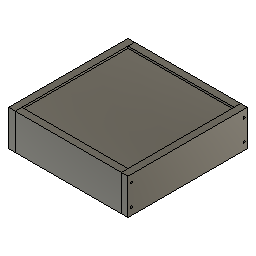
frame_16x16 (Autodesk Fusion 360 design; units mm, degrees)
Autodesk Fusion 360 part; units mm, degrees
note: some values were not read from the file. Set by a fixed rule: which sketch regions a step uses.
(part 1 of 4)
sketch "Sketch1" plane through (0, 0, 0) normal (0, 0, 1) x (1, 0, 0) in component "LED_Pannel"
  line L0 (0, 0) -> (160, 0)
  line L1 (160, 0) -> (160, 160)
  line L2 (160, 160) -> (0, 160)
  line L3 (0, 160) -> (0, 0)
  dimension "d1" = 160
  dimension "d2" = 160
  constraint horizontal L0
  constraint vertical L1
  constraint horizontal L2
  constraint vertical L3
  constraint coincident L0.start L3.end
  measures "d1" distance of L0.start L0.end
  measures "d2" distance of L0.start L2.end
extrude "Extrude1" add sketch "Sketch1" along normal blind 0.2 makes body 1 in component "LED_Pannel"
sketch "Sketch2" plane through (0, 0, 0.2) normal (0, 0, 1) x (-1, 0, 0) in component "LED_Pannel"
  line L0 (0, -160) -> (0, 0)
  line L1 (0, 0) -> (-160, 0)
  line L2 (-160, 0) -> (-160, -160)
  line L3 (-160, -160) -> (0, -160)
  line L4 (-2.5, -2.5) -> (-7.5, -2.5)
  line L5 (-7.5, -2.5) -> (-7.5, -7.5)
  line L6 (-7.5, -7.5) -> (-2.5, -7.5)
  line L7 (-2.5, -7.5) -> (-2.5, -2.5)
  line L8 (-12.5, -7.5) -> (-12.5, -2.5)
  line L9 (-17.5, -7.5) -> (-12.5, -7.5)
  line L10 (-17.5, -2.5) -> (-17.5, -7.5)
  line L11 (-12.5, -2.5) -> (-17.5, -2.5)
  line L12 (-22.5, -7.5) -> (-22.5, -2.5)
  line L13 (-27.5, -7.5) -> (-22.5, -7.5)
  line L14 (-27.5, -2.5) -> (-27.5, -7.5)
  line L15 (-22.5, -2.5) -> (-27.5, -2.5)
  line L16 (-32.5, -7.5) -> (-32.5, -2.5)
  line L17 (-37.5, -7.5) -> (-32.5, -7.5)
  line L18 (-37.5, -2.5) -> (-37.5, -7.5)
  line L19 (-32.5, -2.5) -> (-37.5, -2.5)
  line L20 (-42.5, -7.5) -> (-42.5, -2.5)
  line L21 (-47.5, -7.5) -> (-42.5, -7.5)
  line L22 (-47.5, -2.5) -> (-47.5, -7.5)
  line L23 (-42.5, -2.5) -> (-47.5, -2.5)
  line L24 (-52.5, -7.5) -> (-52.5, -2.5)
  line L25 (-57.5, -7.5) -> (-52.5, -7.5)
  line L26 (-57.5, -2.5) -> (-57.5, -7.5)
  line L27 (-52.5, -2.5) -> (-57.5, -2.5)
  line L28 (-62.5, -7.5) -> (-62.5, -2.5)
  line L29 (-67.5, -7.5) -> (-62.5, -7.5)
  line L30 (-67.5, -2.5) -> (-67.5, -7.5)
  line L31 (-62.5, -2.5) -> (-67.5, -2.5)
  line L32 (-72.5, -7.5) -> (-72.5, -2.5)
  line L33 (-77.5, -7.5) -> (-72.5, -7.5)
  line L34 (-77.5, -2.5) -> (-77.5, -7.5)
  line L35 (-72.5, -2.5) -> (-77.5, -2.5)
  line L36 (-82.5, -7.5) -> (-82.5, -2.5)
  line L37 (-87.5, -7.5) -> (-82.5, -7.5)
  line L38 (-87.5, -2.5) -> (-87.5, -7.5)
  line L39 (-82.5, -2.5) -> (-87.5, -2.5)
  line L40 (-92.5, -7.5) -> (-92.5, -2.5)
  line L41 (-97.5, -7.5) -> (-92.5, -7.5)
  line L42 (-97.5, -2.5) -> (-97.5, -7.5)
  line L43 (-92.5, -2.5) -> (-97.5, -2.5)
  line L44 (-102.5, -7.5) -> (-102.5, -2.5)
  line L45 (-107.5, -7.5) -> (-102.5, -7.5)
  line L46 (-107.5, -2.5) -> (-107.5, -7.5)
  line L47 (-102.5, -2.5) -> (-107.5, -2.5)
  line L48 (-112.5, -7.5) -> (-112.5, -2.5)
  line L49 (-117.5, -7.5) -> (-112.5, -7.5)
  line L50 (-117.5, -2.5) -> (-117.5, -7.5)
  line L51 (-112.5, -2.5) -> (-117.5, -2.5)
  line L52 (-122.5, -7.5) -> (-122.5, -2.5)
  line L53 (-127.5, -7.5) -> (-122.5, -7.5)
  line L54 (-127.5, -2.5) -> (-127.5, -7.5)
  line L55 (-122.5, -2.5) -> (-127.5, -2.5)
  line L56 (-132.5, -7.5) -> (-132.5, -2.5)
  line L57 (-137.5, -7.5) -> (-132.5, -7.5)
  line L58 (-137.5, -2.5) -> (-137.5, -7.5)
  line L59 (-132.5, -2.5) -> (-137.5, -2.5)
  line L60 (-142.5, -7.5) -> (-142.5, -2.5)
  line L61 (-147.5, -7.5) -> (-142.5, -7.5)
  line L62 (-147.5, -2.5) -> (-147.5, -7.5)
  line L63 (-142.5, -2.5) -> (-147.5, -2.5)
  line L64 (-152.5, -7.5) -> (-152.5, -2.5)
  line L65 (-157.5, -7.5) -> (-152.5, -7.5)
  line L66 (-157.5, -2.5) -> (-157.5, -7.5)
  line L67 (-152.5, -2.5) -> (-157.5, -2.5)
  line L68 (-2.5, -17.5) -> (-2.5, -12.5)
  line L69 (-7.5, -17.5) -> (-2.5, -17.5)
  line L70 (-7.5, -12.5) -> (-7.5, -17.5)
  line L71 (-2.5, -12.5) -> (-7.5, -12.5)
  line L72 (-12.5, -17.5) -> (-12.5, -12.5)
  line L73 (-17.5, -17.5) -> (-12.5, -17.5)
  line L74 (-17.5, -12.5) -> (-17.5, -17.5)
  line L75 (-12.5, -12.5) -> (-17.5, -12.5)
  line L76 (-22.5, -17.5) -> (-22.5, -12.5)
  line L77 (-27.5, -17.5) -> (-22.5, -17.5)
  line L78 (-27.5, -12.5) -> (-27.5, -17.5)
  line L79 (-22.5, -12.5) -> (-27.5, -12.5)
  line L80 (-32.5, -17.5) -> (-32.5, -12.5)
  line L81 (-37.5, -17.5) -> (-32.5, -17.5)
  line L82 (-37.5, -12.5) -> (-37.5, -17.5)
  line L83 (-32.5, -12.5) -> (-37.5, -12.5)
  line L84 (-42.5, -17.5) -> (-42.5, -12.5)
  line L85 (-47.5, -17.5) -> (-42.5, -17.5)
  line L86 (-47.5, -12.5) -> (-47.5, -17.5)
  line L87 (-42.5, -12.5) -> (-47.5, -12.5)
  line L88 (-52.5, -17.5) -> (-52.5, -12.5)
  line L89 (-57.5, -17.5) -> (-52.5, -17.5)
  line L90 (-57.5, -12.5) -> (-57.5, -17.5)
  line L91 (-52.5, -12.5) -> (-57.5, -12.5)
  line L92 (-62.5, -17.5) -> (-62.5, -12.5)
  line L93 (-67.5, -17.5) -> (-62.5, -17.5)
  line L94 (-67.5, -12.5) -> (-67.5, -17.5)
  line L95 (-62.5, -12.5) -> (-67.5, -12.5)
  line L96 (-72.5, -17.5) -> (-72.5, -12.5)
  line L97 (-77.5, -17.5) -> (-72.5, -17.5)
  line L98 (-77.5, -12.5) -> (-77.5, -17.5)
  line L99 (-72.5, -12.5) -> (-77.5, -12.5)
  line L100 (-82.5, -17.5) -> (-82.5, -12.5)
  line L101 (-87.5, -17.5) -> (-82.5, -17.5)
  line L102 (-87.5, -12.5) -> (-87.5, -17.5)
  line L103 (-82.5, -12.5) -> (-87.5, -12.5)
  line L104 (-92.5, -17.5) -> (-92.5, -12.5)
  line L105 (-97.5, -17.5) -> (-92.5, -17.5)
  line L106 (-97.5, -12.5) -> (-97.5, -17.5)
  line L107 (-92.5, -12.5) -> (-97.5, -12.5)
  line L108 (-102.5, -17.5) -> (-102.5, -12.5)
  line L109 (-107.5, -17.5) -> (-102.5, -17.5)
  line L110 (-107.5, -12.5) -> (-107.5, -17.5)
  line L111 (-102.5, -12.5) -> (-107.5, -12.5)
  line L112 (-112.5, -17.5) -> (-112.5, -12.5)
  line L113 (-117.5, -17.5) -> (-112.5, -17.5)
  line L114 (-117.5, -12.5) -> (-117.5, -17.5)
  line L115 (-112.5, -12.5) -> (-117.5, -12.5)
  line L116 (-122.5, -17.5) -> (-122.5, -12.5)
  line L117 (-127.5, -17.5) -> (-122.5, -17.5)
  line L118 (-127.5, -12.5) -> (-127.5, -17.5)
  line L119 (-122.5, -12.5) -> (-127.5, -12.5)
  line L120 (-132.5, -17.5) -> (-132.5, -12.5)
  line L121 (-137.5, -17.5) -> (-132.5, -17.5)
  line L122 (-137.5, -12.5) -> (-137.5, -17.5)
  line L123 (-132.5, -12.5) -> (-137.5, -12.5)
  line L124 (-142.5, -17.5) -> (-142.5, -12.5)
  line L125 (-147.5, -17.5) -> (-142.5, -17.5)
  line L126 (-147.5, -12.5) -> (-147.5, -17.5)
  line L127 (-142.5, -12.5) -> (-147.5, -12.5)
  line L128 (-152.5, -17.5) -> (-152.5, -12.5)
  line L129 (-157.5, -17.5) -> (-152.5, -17.5)
  line L130 (-157.5, -12.5) -> (-157.5, -17.5)
  line L131 (-152.5, -12.5) -> (-157.5, -12.5)
  line L132 (-2.5, -27.5) -> (-2.5, -22.5)
  line L133 (-7.5, -27.5) -> (-2.5, -27.5)
  line L134 (-7.5, -22.5) -> (-7.5, -27.5)
  line L135 (-2.5, -22.5) -> (-7.5, -22.5)
  line L136 (-12.5, -27.5) -> (-12.5, -22.5)
  line L137 (-17.5, -27.5) -> (-12.5, -27.5)
  line L138 (-17.5, -22.5) -> (-17.5, -27.5)
  line L139 (-12.5, -22.5) -> (-17.5, -22.5)
  line L140 (-22.5, -27.5) -> (-22.5, -22.5)
  line L141 (-27.5, -27.5) -> (-22.5, -27.5)
  line L142 (-27.5, -22.5) -> (-27.5, -27.5)
  line L143 (-22.5, -22.5) -> (-27.5, -22.5)
  line L144 (-32.5, -27.5) -> (-32.5, -22.5)
  line L145 (-37.5, -27.5) -> (-32.5, -27.5)
  line L146 (-37.5, -22.5) -> (-37.5, -27.5)
  line L147 (-32.5, -22.5) -> (-37.5, -22.5)
  line L148 (-42.5, -27.5) -> (-42.5, -22.5)
  line L149 (-47.5, -27.5) -> (-42.5, -27.5)
  line L150 (-47.5, -22.5) -> (-47.5, -27.5)
  line L151 (-42.5, -22.5) -> (-47.5, -22.5)
  line L152 (-52.5, -27.5) -> (-52.5, -22.5)
  line L153 (-57.5, -27.5) -> (-52.5, -27.5)
  line L154 (-57.5, -22.5) -> (-57.5, -27.5)
  line L155 (-52.5, -22.5) -> (-57.5, -22.5)
  line L156 (-62.5, -27.5) -> (-62.5, -22.5)
  line L157 (-67.5, -27.5) -> (-62.5, -27.5)
  line L158 (-67.5, -22.5) -> (-67.5, -27.5)
  line L159 (-62.5, -22.5) -> (-67.5, -22.5)
  line L160 (-72.5, -27.5) -> (-72.5, -22.5)
  line L161 (-77.5, -27.5) -> (-72.5, -27.5)
  line L162 (-77.5, -22.5) -> (-77.5, -27.5)
  line L163 (-72.5, -22.5) -> (-77.5, -22.5)
  line L164 (-82.5, -27.5) -> (-82.5, -22.5)
  line L165 (-87.5, -27.5) -> (-82.5, -27.5)
  line L166 (-87.5, -22.5) -> (-87.5, -27.5)
  line L167 (-82.5, -22.5) -> (-87.5, -22.5)
  line L168 (-92.5, -27.5) -> (-92.5, -22.5)
  line L169 (-97.5, -27.5) -> (-92.5, -27.5)
  line L170 (-97.5, -22.5) -> (-97.5, -27.5)
  line L171 (-92.5, -22.5) -> (-97.5, -22.5)
  line L172 (-102.5, -27.5) -> (-102.5, -22.5)
  line L173 (-107.5, -27.5) -> (-102.5, -27.5)
  line L174 (-107.5, -22.5) -> (-107.5, -27.5)
  line L175 (-102.5, -22.5) -> (-107.5, -22.5)
  line L176 (-112.5, -27.5) -> (-112.5, -22.5)
  line L177 (-117.5, -27.5) -> (-112.5, -27.5)
  line L178 (-117.5, -22.5) -> (-117.5, -27.5)
  line L179 (-112.5, -22.5) -> (-117.5, -22.5)
  line L180 (-122.5, -27.5) -> (-122.5, -22.5)
  line L181 (-127.5, -27.5) -> (-122.5, -27.5)
  line L182 (-127.5, -22.5) -> (-127.5, -27.5)
  line L183 (-122.5, -22.5) -> (-127.5, -22.5)
  line L184 (-132.5, -27.5) -> (-132.5, -22.5)
  line L185 (-137.5, -27.5) -> (-132.5, -27.5)
  line L186 (-137.5, -22.5) -> (-137.5, -27.5)
  line L187 (-132.5, -22.5) -> (-137.5, -22.5)
  line L188 (-142.5, -27.5) -> (-142.5, -22.5)
  line L189 (-147.5, -27.5) -> (-142.5, -27.5)
  line L190 (-147.5, -22.5) -> (-147.5, -27.5)
  line L191 (-142.5, -22.5) -> (-147.5, -22.5)
  line L192 (-152.5, -27.5) -> (-152.5, -22.5)
  line L193 (-157.5, -27.5) -> (-152.5, -27.5)
  line L194 (-157.5, -22.5) -> (-157.5, -27.5)
  line L195 (-152.5, -22.5) -> (-157.5, -22.5)
  line L196 (-2.5, -37.5) -> (-2.5, -32.5)
  line L197 (-7.5, -37.5) -> (-2.5, -37.5)
  line L198 (-7.5, -32.5) -> (-7.5, -37.5)
  line L199 (-2.5, -32.5) -> (-7.5, -32.5)
  line L200 (-12.5, -37.5) -> (-12.5, -32.5)
  line L201 (-17.5, -37.5) -> (-12.5, -37.5)
  line L202 (-17.5, -32.5) -> (-17.5, -37.5)
  line L203 (-12.5, -32.5) -> (-17.5, -32.5)
  line L204 (-22.5, -37.5) -> (-22.5, -32.5)
  line L205 (-27.5, -37.5) -> (-22.5, -37.5)
  line L206 (-27.5, -32.5) -> (-27.5, -37.5)
  line L207 (-22.5, -32.5) -> (-27.5, -32.5)
  line L208 (-32.5, -37.5) -> (-32.5, -32.5)
  line L209 (-37.5, -37.5) -> (-32.5, -37.5)
  line L210 (-37.5, -32.5) -> (-37.5, -37.5)
  line L211 (-32.5, -32.5) -> (-37.5, -32.5)
  line L212 (-42.5, -37.5) -> (-42.5, -32.5)
  line L213 (-47.5, -37.5) -> (-42.5, -37.5)
  line L214 (-47.5, -32.5) -> (-47.5, -37.5)
  line L215 (-42.5, -32.5) -> (-47.5, -32.5)
  line L216 (-52.5, -37.5) -> (-52.5, -32.5)
  line L217 (-57.5, -37.5) -> (-52.5, -37.5)
  line L218 (-57.5, -32.5) -> (-57.5, -37.5)
  line L219 (-52.5, -32.5) -> (-57.5, -32.5)
  line L220 (-62.5, -37.5) -> (-62.5, -32.5)
  line L221 (-67.5, -37.5) -> (-62.5, -37.5)
  line L222 (-67.5, -32.5) -> (-67.5, -37.5)
  line L223 (-62.5, -32.5) -> (-67.5, -32.5)
  line L224 (-72.5, -37.5) -> (-72.5, -32.5)
  line L225 (-77.5, -37.5) -> (-72.5, -37.5)
  line L226 (-77.5, -32.5) -> (-77.5, -37.5)
  line L227 (-72.5, -32.5) -> (-77.5, -32.5)
  line L228 (-82.5, -37.5) -> (-82.5, -32.5)
  line L229 (-87.5, -37.5) -> (-82.5, -37.5)
  line L230 (-87.5, -32.5) -> (-87.5, -37.5)
  line L231 (-82.5, -32.5) -> (-87.5, -32.5)
  line L232 (-92.5, -37.5) -> (-92.5, -32.5)
  line L233 (-97.5, -37.5) -> (-92.5, -37.5)
  line L234 (-97.5, -32.5) -> (-97.5, -37.5)
  line L235 (-92.5, -32.5) -> (-97.5, -32.5)
  line L236 (-102.5, -37.5) -> (-102.5, -32.5)
  line L237 (-107.5, -37.5) -> (-102.5, -37.5)
  line L238 (-107.5, -32.5) -> (-107.5, -37.5)
  line L239 (-102.5, -32.5) -> (-107.5, -32.5)
  line L240 (-112.5, -37.5) -> (-112.5, -32.5)
  line L241 (-117.5, -37.5) -> (-112.5, -37.5)
  line L242 (-117.5, -32.5) -> (-117.5, -37.5)
  line L243 (-112.5, -32.5) -> (-117.5, -32.5)
  line L244 (-122.5, -37.5) -> (-122.5, -32.5)
  line L245 (-127.5, -37.5) -> (-122.5, -37.5)
  line L246 (-127.5, -32.5) -> (-127.5, -37.5)
  line L247 (-122.5, -32.5) -> (-127.5, -32.5)
  line L248 (-132.5, -37.5) -> (-132.5, -32.5)
  line L249 (-137.5, -37.5) -> (-132.5, -37.5)
  line L250 (-137.5, -32.5) -> (-137.5, -37.5)
  line L251 (-132.5, -32.5) -> (-137.5, -32.5)
  line L252 (-142.5, -37.5) -> (-142.5, -32.5)
  line L253 (-147.5, -37.5) -> (-142.5, -37.5)
  line L254 (-147.5, -32.5) -> (-147.5, -37.5)
  line L255 (-142.5, -32.5) -> (-147.5, -32.5)
  line L256 (-152.5, -37.5) -> (-152.5, -32.5)
  line L257 (-157.5, -37.5) -> (-152.5, -37.5)
  line L258 (-157.5, -32.5) -> (-157.5, -37.5)
  line L259 (-152.5, -32.5) -> (-157.5, -32.5)
  line L260 (-2.5, -47.5) -> (-2.5, -42.5)
  line L261 (-7.5, -47.5) -> (-2.5, -47.5)
  line L262 (-7.5, -42.5) -> (-7.5, -47.5)
  line L263 (-2.5, -42.5) -> (-7.5, -42.5)
  line L264 (-12.5, -47.5) -> (-12.5, -42.5)
  line L265 (-17.5, -47.5) -> (-12.5, -47.5)
  line L266 (-17.5, -42.5) -> (-17.5, -47.5)
  line L267 (-12.5, -42.5) -> (-17.5, -42.5)
  line L268 (-22.5, -47.5) -> (-22.5, -42.5)
  line L269 (-27.5, -47.5) -> (-22.5, -47.5)
  line L270 (-27.5, -42.5) -> (-27.5, -47.5)
  line L271 (-22.5, -42.5) -> (-27.5, -42.5)
  line L272 (-32.5, -47.5) -> (-32.5, -42.5)
  line L273 (-37.5, -47.5) -> (-32.5, -47.5)
  line L274 (-37.5, -42.5) -> (-37.5, -47.5)
  line L275 (-32.5, -42.5) -> (-37.5, -42.5)
  line L276 (-42.5, -47.5) -> (-42.5, -42.5)
  line L277 (-47.5, -47.5) -> (-42.5, -47.5)
  line L278 (-47.5, -42.5) -> (-47.5, -47.5)
  line L279 (-42.5, -42.5) -> (-47.5, -42.5)
  line L280 (-52.5, -47.5) -> (-52.5, -42.5)
  line L281 (-57.5, -47.5) -> (-52.5, -47.5)
  line L282 (-57.5, -42.5) -> (-57.5, -47.5)
  line L283 (-52.5, -42.5) -> (-57.5, -42.5)
  line L284 (-62.5, -47.5) -> (-62.5, -42.5)
  line L285 (-67.5, -47.5) -> (-62.5, -47.5)
  line L286 (-67.5, -42.5) -> (-67.5, -47.5)
  line L287 (-62.5, -42.5) -> (-67.5, -42.5)
  line L288 (-72.5, -47.5) -> (-72.5, -42.5)
  line L289 (-77.5, -47.5) -> (-72.5, -47.5)
  line L290 (-77.5, -42.5) -> (-77.5, -47.5)
  line L291 (-72.5, -42.5) -> (-77.5, -42.5)
  line L292 (-82.5, -47.5) -> (-82.5, -42.5)
  line L293 (-87.5, -47.5) -> (-82.5, -47.5)
  line L294 (-87.5, -42.5) -> (-87.5, -47.5)
  line L295 (-82.5, -42.5) -> (-87.5, -42.5)
  line L296 (-92.5, -47.5) -> (-92.5, -42.5)
  line L297 (-97.5, -47.5) -> (-92.5, -47.5)
  line L298 (-97.5, -42.5) -> (-97.5, -47.5)
  line L299 (-92.5, -42.5) -> (-97.5, -42.5)
  line L300 (-102.5, -47.5) -> (-102.5, -42.5)
  line L301 (-107.5, -47.5) -> (-102.5, -47.5)
  line L302 (-107.5, -42.5) -> (-107.5, -47.5)
  line L303 (-102.5, -42.5) -> (-107.5, -42.5)
  line L304 (-112.5, -47.5) -> (-112.5, -42.5)
  line L305 (-117.5, -47.5) -> (-112.5, -47.5)
  line L306 (-117.5, -42.5) -> (-117.5, -47.5)
  line L307 (-112.5, -42.5) -> (-117.5, -42.5)
  line L308 (-122.5, -47.5) -> (-122.5, -42.5)
  line L309 (-127.5, -47.5) -> (-122.5, -47.5)
  line L310 (-127.5, -42.5) -> (-127.5, -47.5)
  line L311 (-122.5, -42.5) -> (-127.5, -42.5)
  line L312 (-132.5, -47.5) -> (-132.5, -42.5)
  line L313 (-137.5, -47.5) -> (-132.5, -47.5)
  line L314 (-137.5, -42.5) -> (-137.5, -47.5)
  line L315 (-132.5, -42.5) -> (-137.5, -42.5)
  line L316 (-142.5, -47.5) -> (-142.5, -42.5)
  line L317 (-147.5, -47.5) -> (-142.5, -47.5)
  line L318 (-147.5, -42.5) -> (-147.5, -47.5)
  line L319 (-142.5, -42.5) -> (-147.5, -42.5)
  line L320 (-152.5, -47.5) -> (-152.5, -42.5)
  line L321 (-157.5, -47.5) -> (-152.5, -47.5)
  line L322 (-157.5, -42.5) -> (-157.5, -47.5)
  line L323 (-152.5, -42.5) -> (-157.5, -42.5)
  line L324 (-2.5, -57.5) -> (-2.5, -52.5)
  line L325 (-7.5, -57.5) -> (-2.5, -57.5)
  line L326 (-7.5, -52.5) -> (-7.5, -57.5)
  line L327 (-2.5, -52.5) -> (-7.5, -52.5)
  line L328 (-12.5, -57.5) -> (-12.5, -52.5)
  line L329 (-17.5, -57.5) -> (-12.5, -57.5)
  line L330 (-17.5, -52.5) -> (-17.5, -57.5)
  line L331 (-12.5, -52.5) -> (-17.5, -52.5)
  line L332 (-22.5, -57.5) -> (-22.5, -52.5)
  line L333 (-27.5, -57.5) -> (-22.5, -57.5)
  line L334 (-27.5, -52.5) -> (-27.5, -57.5)
  line L335 (-22.5, -52.5) -> (-27.5, -52.5)
  line L336 (-32.5, -57.5) -> (-32.5, -52.5)
  line L337 (-37.5, -57.5) -> (-32.5, -57.5)
  line L338 (-37.5, -52.5) -> (-37.5, -57.5)
  line L339 (-32.5, -52.5) -> (-37.5, -52.5)
  line L340 (-42.5, -57.5) -> (-42.5, -52.5)
  line L341 (-47.5, -57.5) -> (-42.5, -57.5)
  line L342 (-47.5, -52.5) -> (-47.5, -57.5)
  line L343 (-42.5, -52.5) -> (-47.5, -52.5)
  line L344 (-52.5, -57.5) -> (-52.5, -52.5)
  line L345 (-57.5, -57.5) -> (-52.5, -57.5)
  line L346 (-57.5, -52.5) -> (-57.5, -57.5)
  line L347 (-52.5, -52.5) -> (-57.5, -52.5)
  line L348 (-62.5, -57.5) -> (-62.5, -52.5)
  line L349 (-67.5, -57.5) -> (-62.5, -57.5)
  line L350 (-67.5, -52.5) -> (-67.5, -57.5)
  line L351 (-62.5, -52.5) -> (-67.5, -52.5)
  line L352 (-72.5, -57.5) -> (-72.5, -52.5)
  line L353 (-77.5, -57.5) -> (-72.5, -57.5)
  line L354 (-77.5, -52.5) -> (-77.5, -57.5)
  line L355 (-72.5, -52.5) -> (-77.5, -52.5)
  line L356 (-82.5, -57.5) -> (-82.5, -52.5)
  line L357 (-87.5, -57.5) -> (-82.5, -57.5)
  line L358 (-87.5, -52.5) -> (-87.5, -57.5)
  line L359 (-82.5, -52.5) -> (-87.5, -52.5)
  line L360 (-92.5, -57.5) -> (-92.5, -52.5)
  line L361 (-97.5, -57.5) -> (-92.5, -57.5)
  line L362 (-97.5, -52.5) -> (-97.5, -57.5)
  line L363 (-92.5, -52.5) -> (-97.5, -52.5)
  line L364 (-102.5, -57.5) -> (-102.5, -52.5)
  line L365 (-107.5, -57.5) -> (-102.5, -57.5)
  line L366 (-107.5, -52.5) -> (-107.5, -57.5)
  line L367 (-102.5, -52.5) -> (-107.5, -52.5)
  line L368 (-112.5, -57.5) -> (-112.5, -52.5)
  line L369 (-117.5, -57.5) -> (-112.5, -57.5)
  line L370 (-117.5, -52.5) -> (-117.5, -57.5)
  line L371 (-112.5, -52.5) -> (-117.5, -52.5)
  line L372 (-122.5, -57.5) -> (-122.5, -52.5)
  line L373 (-127.5, -57.5) -> (-122.5, -57.5)
  line L374 (-127.5, -52.5) -> (-127.5, -57.5)
  line L375 (-122.5, -52.5) -> (-127.5, -52.5)
  line L376 (-132.5, -57.5) -> (-132.5, -52.5)
  line L377 (-137.5, -57.5) -> (-132.5, -57.5)
  line L378 (-137.5, -52.5) -> (-137.5, -57.5)
  line L379 (-132.5, -52.5) -> (-137.5, -52.5)
  line L380 (-142.5, -57.5) -> (-142.5, -52.5)
  line L381 (-147.5, -57.5) -> (-142.5, -57.5)
  line L382 (-147.5, -52.5) -> (-147.5, -57.5)
  line L383 (-142.5, -52.5) -> (-147.5, -52.5)
  line L384 (-152.5, -57.5) -> (-152.5, -52.5)
  line L385 (-157.5, -57.5) -> (-152.5, -57.5)
  line L386 (-157.5, -52.5) -> (-157.5, -57.5)
  line L387 (-152.5, -52.5) -> (-157.5, -52.5)
  line L388 (-2.5, -67.5) -> (-2.5, -62.5)
  line L389 (-7.5, -67.5) -> (-2.5, -67.5)
  line L390 (-7.5, -62.5) -> (-7.5, -67.5)
  line L391 (-2.5, -62.5) -> (-7.5, -62.5)
  line L392 (-12.5, -67.5) -> (-12.5, -62.5)
  line L393 (-17.5, -67.5) -> (-12.5, -67.5)
  line L394 (-17.5, -62.5) -> (-17.5, -67.5)
  line L395 (-12.5, -62.5) -> (-17.5, -62.5)
  line L396 (-22.5, -67.5) -> (-22.5, -62.5)
  line L397 (-27.5, -67.5) -> (-22.5, -67.5)
  line L398 (-27.5, -62.5) -> (-27.5, -67.5)
  line L399 (-22.5, -62.5) -> (-27.5, -62.5)
  line L400 (-32.5, -67.5) -> (-32.5, -62.5)
  line L401 (-37.5, -67.5) -> (-32.5, -67.5)
  line L402 (-37.5, -62.5) -> (-37.5, -67.5)
  line L403 (-32.5, -62.5) -> (-37.5, -62.5)
  line L404 (-42.5, -67.5) -> (-42.5, -62.5)
  line L405 (-47.5, -67.5) -> (-42.5, -67.5)
  line L406 (-47.5, -62.5) -> (-47.5, -67.5)
  line L407 (-42.5, -62.5) -> (-47.5, -62.5)
  line L408 (-52.5, -67.5) -> (-52.5, -62.5)
  line L409 (-57.5, -67.5) -> (-52.5, -67.5)
  line L410 (-57.5, -62.5) -> (-57.5, -67.5)
  line L411 (-52.5, -62.5) -> (-57.5, -62.5)
  line L412 (-62.5, -67.5) -> (-62.5, -62.5)
  line L413 (-67.5, -67.5) -> (-62.5, -67.5)
  line L414 (-67.5, -62.5) -> (-67.5, -67.5)
  line L415 (-62.5, -62.5) -> (-67.5, -62.5)
  line L416 (-72.5, -67.5) -> (-72.5, -62.5)
  line L417 (-77.5, -67.5) -> (-72.5, -67.5)
  line L418 (-77.5, -62.5) -> (-77.5, -67.5)
  line L419 (-72.5, -62.5) -> (-77.5, -62.5)
  line L420 (-82.5, -67.5) -> (-82.5, -62.5)
  line L421 (-87.5, -67.5) -> (-82.5, -67.5)
  line L422 (-87.5, -62.5) -> (-87.5, -67.5)
  line L423 (-82.5, -62.5) -> (-87.5, -62.5)
  line L424 (-92.5, -67.5) -> (-92.5, -62.5)
  line L425 (-97.5, -67.5) -> (-92.5, -67.5)
  line L426 (-97.5, -62.5) -> (-97.5, -67.5)
  line L427 (-92.5, -62.5) -> (-97.5, -62.5)
  line L428 (-102.5, -67.5) -> (-102.5, -62.5)
  line L429 (-107.5, -67.5) -> (-102.5, -67.5)
  line L430 (-107.5, -62.5) -> (-107.5, -67.5)
  line L431 (-102.5, -62.5) -> (-107.5, -62.5)
  line L432 (-112.5, -67.5) -> (-112.5, -62.5)
  line L433 (-117.5, -67.5) -> (-112.5, -67.5)
  line L434 (-117.5, -62.5) -> (-117.5, -67.5)
  line L435 (-112.5, -62.5) -> (-117.5, -62.5)
  line L436 (-122.5, -67.5) -> (-122.5, -62.5)
  line L437 (-127.5, -67.5) -> (-122.5, -67.5)
  line L438 (-127.5, -62.5) -> (-127.5, -67.5)
  line L439 (-122.5, -62.5) -> (-127.5, -62.5)
  line L440 (-132.5, -67.5) -> (-132.5, -62.5)
  line L441 (-137.5, -67.5) -> (-132.5, -67.5)
  line L442 (-137.5, -62.5) -> (-137.5, -67.5)
  line L443 (-132.5, -62.5) -> (-137.5, -62.5)
  line L444 (-142.5, -67.5) -> (-142.5, -62.5)
  line L445 (-147.5, -67.5) -> (-142.5, -67.5)
  line L446 (-147.5, -62.5) -> (-147.5, -67.5)
  line L447 (-142.5, -62.5) -> (-147.5, -62.5)
  line L448 (-152.5, -67.5) -> (-152.5, -62.5)
  line L449 (-157.5, -67.5) -> (-152.5, -67.5)
  line L450 (-157.5, -62.5) -> (-157.5, -67.5)
  line L451 (-152.5, -62.5) -> (-157.5, -62.5)
  line L452 (-2.5, -77.5) -> (-2.5, -72.5)
  line L453 (-7.5, -77.5) -> (-2.5, -77.5)
  line L454 (-7.5, -72.5) -> (-7.5, -77.5)
  line L455 (-2.5, -72.5) -> (-7.5, -72.5)
  line L456 (-12.5, -77.5) -> (-12.5, -72.5)
  line L457 (-17.5, -77.5) -> (-12.5, -77.5)
  line L458 (-17.5, -72.5) -> (-17.5, -77.5)
  line L459 (-12.5, -72.5) -> (-17.5, -72.5)
  line L460 (-22.5, -77.5) -> (-22.5, -72.5)
  line L461 (-27.5, -77.5) -> (-22.5, -77.5)
  line L462 (-27.5, -72.5) -> (-27.5, -77.5)
  line L463 (-22.5, -72.5) -> (-27.5, -72.5)
  line L464 (-32.5, -77.5) -> (-32.5, -72.5)
  line L465 (-37.5, -77.5) -> (-32.5, -77.5)
  line L466 (-37.5, -72.5) -> (-37.5, -77.5)
  line L467 (-32.5, -72.5) -> (-37.5, -72.5)
  line L468 (-42.5, -77.5) -> (-42.5, -72.5)
  line L469 (-47.5, -77.5) -> (-42.5, -77.5)
  line L470 (-47.5, -72.5) -> (-47.5, -77.5)
  line L471 (-42.5, -72.5) -> (-47.5, -72.5)
  line L472 (-52.5, -77.5) -> (-52.5, -72.5)
  line L473 (-57.5, -77.5) -> (-52.5, -77.5)
  line L474 (-57.5, -72.5) -> (-57.5, -77.5)
  line L475 (-52.5, -72.5) -> (-57.5, -72.5)
  line L476 (-62.5, -77.5) -> (-62.5, -72.5)
  line L477 (-67.5, -77.5) -> (-62.5, -77.5)
  line L478 (-67.5, -72.5) -> (-67.5, -77.5)
  line L479 (-62.5, -72.5) -> (-67.5, -72.5)
  line L480 (-72.5, -77.5) -> (-72.5, -72.5)
  line L481 (-77.5, -77.5) -> (-72.5, -77.5)
  line L482 (-77.5, -72.5) -> (-77.5, -77.5)
  line L483 (-72.5, -72.5) -> (-77.5, -72.5)
  line L484 (-82.5, -77.5) -> (-82.5, -72.5)
  line L485 (-87.5, -77.5) -> (-82.5, -77.5)
  line L486 (-87.5, -72.5) -> (-87.5, -77.5)
  line L487 (-82.5, -72.5) -> (-87.5, -72.5)
  line L488 (-92.5, -77.5) -> (-92.5, -72.5)
  line L489 (-97.5, -77.5) -> (-92.5, -77.5)
  line L490 (-97.5, -72.5) -> (-97.5, -77.5)
  line L491 (-92.5, -72.5) -> (-97.5, -72.5)
  line L492 (-102.5, -77.5) -> (-102.5, -72.5)
  line L493 (-107.5, -77.5) -> (-102.5, -77.5)
  line L494 (-107.5, -72.5) -> (-107.5, -77.5)
  line L495 (-102.5, -72.5) -> (-107.5, -72.5)
  line L496 (-112.5, -77.5) -> (-112.5, -72.5)
  line L497 (-117.5, -77.5) -> (-112.5, -77.5)
  line L498 (-117.5, -72.5) -> (-117.5, -77.5)
  line L499 (-112.5, -72.5) -> (-117.5, -72.5)
  line L500 (-122.5, -77.5) -> (-122.5, -72.5)
  line L501 (-127.5, -77.5) -> (-122.5, -77.5)
  line L502 (-127.5, -72.5) -> (-127.5, -77.5)
  line L503 (-122.5, -72.5) -> (-127.5, -72.5)
  line L504 (-132.5, -77.5) -> (-132.5, -72.5)
  line L505 (-137.5, -77.5) -> (-132.5, -77.5)
  line L506 (-137.5, -72.5) -> (-137.5, -77.5)
  line L507 (-132.5, -72.5) -> (-137.5, -72.5)
  line L508 (-142.5, -77.5) -> (-142.5, -72.5)
  line L509 (-147.5, -77.5) -> (-142.5, -77.5)
  line L510 (-147.5, -72.5) -> (-147.5, -77.5)
  line L511 (-142.5, -72.5) -> (-147.5, -72.5)
  line L512 (-152.5, -77.5) -> (-152.5, -72.5)
  line L513 (-157.5, -77.5) -> (-152.5, -77.5)
  line L514 (-157.5, -72.5) -> (-157.5, -77.5)
  line L515 (-152.5, -72.5) -> (-157.5, -72.5)
  line L516 (-2.5, -87.5) -> (-2.5, -82.5)
  line L517 (-7.5, -87.5) -> (-2.5, -87.5)
  line L518 (-7.5, -82.5) -> (-7.5, -87.5)
  line L519 (-2.5, -82.5) -> (-7.5, -82.5)
  line L520 (-12.5, -87.5) -> (-12.5, -82.5)
  line L521 (-17.5, -87.5) -> (-12.5, -87.5)
  line L522 (-17.5, -82.5) -> (-17.5, -87.5)
  line L523 (-12.5, -82.5) -> (-17.5, -82.5)
  line L524 (-22.5, -87.5) -> (-22.5, -82.5)
  line L525 (-27.5, -87.5) -> (-22.5, -87.5)
  line L526 (-27.5, -82.5) -> (-27.5, -87.5)
  line L527 (-22.5, -82.5) -> (-27.5, -82.5)
  line L528 (-32.5, -87.5) -> (-32.5, -82.5)
  line L529 (-37.5, -87.5) -> (-32.5, -87.5)
  line L530 (-37.5, -82.5) -> (-37.5, -87.5)
  line L531 (-32.5, -82.5) -> (-37.5, -82.5)
  line L532 (-42.5, -87.5) -> (-42.5, -82.5)
  line L533 (-47.5, -87.5) -> (-42.5, -87.5)
  line L534 (-47.5, -82.5) -> (-47.5, -87.5)
  line L535 (-42.5, -82.5) -> (-47.5, -82.5)
  line L536 (-52.5, -87.5) -> (-52.5, -82.5)
  line L537 (-57.5, -87.5) -> (-52.5, -87.5)
  line L538 (-57.5, -82.5) -> (-57.5, -87.5)
  line L539 (-52.5, -82.5) -> (-57.5, -82.5)
  line L540 (-62.5, -87.5) -> (-62.5, -82.5)
  line L541 (-67.5, -87.5) -> (-62.5, -87.5)
  line L542 (-67.5, -82.5) -> (-67.5, -87.5)
  line L543 (-62.5, -82.5) -> (-67.5, -82.5)
  line L544 (-72.5, -87.5) -> (-72.5, -82.5)
  line L545 (-77.5, -87.5) -> (-72.5, -87.5)
  line L546 (-77.5, -82.5) -> (-77.5, -87.5)
  line L547 (-72.5, -82.5) -> (-77.5, -82.5)
  line L548 (-82.5, -87.5) -> (-82.5, -82.5)
  line L549 (-87.5, -87.5) -> (-82.5, -87.5)
  line L550 (-87.5, -82.5) -> (-87.5, -87.5)
  line L551 (-82.5, -82.5) -> (-87.5, -82.5)
  line L552 (-92.5, -87.5) -> (-92.5, -82.5)
  line L553 (-97.5, -87.5) -> (-92.5, -87.5)
  line L554 (-97.5, -82.5) -> (-97.5, -87.5)
  line L555 (-92.5, -82.5) -> (-97.5, -82.5)
  line L556 (-102.5, -87.5) -> (-102.5, -82.5)
  line L557 (-107.5, -87.5) -> (-102.5, -87.5)
  line L558 (-107.5, -82.5) -> (-107.5, -87.5)
  line L559 (-102.5, -82.5) -> (-107.5, -82.5)
  line L560 (-112.5, -87.5) -> (-112.5, -82.5)
  line L561 (-117.5, -87.5) -> (-112.5, -87.5)
  line L562 (-117.5, -82.5) -> (-117.5, -87.5)
  line L563 (-112.5, -82.5) -> (-117.5, -82.5)
  line L564 (-122.5, -87.5) -> (-122.5, -82.5)
  line L565 (-127.5, -87.5) -> (-122.5, -87.5)
  line L566 (-127.5, -82.5) -> (-127.5, -87.5)
  line L567 (-122.5, -82.5) -> (-127.5, -82.5)
  line L568 (-132.5, -87.5) -> (-132.5, -82.5)
  line L569 (-137.5, -87.5) -> (-132.5, -87.5)
  line L570 (-137.5, -82.5) -> (-137.5, -87.5)
  line L571 (-132.5, -82.5) -> (-137.5, -82.5)
  line L572 (-142.5, -87.5) -> (-142.5, -82.5)
  line L573 (-147.5, -87.5) -> (-142.5, -87.5)
  line L574 (-147.5, -82.5) -> (-147.5, -87.5)
  line L575 (-142.5, -82.5) -> (-147.5, -82.5)
  line L576 (-152.5, -87.5) -> (-152.5, -82.5)
  line L577 (-157.5, -87.5) -> (-152.5, -87.5)
  line L578 (-157.5, -82.5) -> (-157.5, -87.5)
  line L579 (-152.5, -82.5) -> (-157.5, -82.5)
  line L580 (-2.5, -97.5) -> (-2.5, -92.5)
  line L581 (-7.5, -97.5) -> (-2.5, -97.5)
  line L582 (-7.5, -92.5) -> (-7.5, -97.5)
  line L583 (-2.5, -92.5) -> (-7.5, -92.5)
  line L584 (-12.5, -97.5) -> (-12.5, -92.5)
  line L585 (-17.5, -97.5) -> (-12.5, -97.5)
  line L586 (-17.5, -92.5) -> (-17.5, -97.5)
  line L587 (-12.5, -92.5) -> (-17.5, -92.5)
  line L588 (-22.5, -97.5) -> (-22.5, -92.5)
  line L589 (-27.5, -97.5) -> (-22.5, -97.5)
  line L590 (-27.5, -92.5) -> (-27.5, -97.5)
  line L591 (-22.5, -92.5) -> (-27.5, -92.5)
  line L592 (-32.5, -97.5) -> (-32.5, -92.5)
  line L593 (-37.5, -97.5) -> (-32.5, -97.5)
  line L594 (-37.5, -92.5) -> (-37.5, -97.5)
  line L595 (-32.5, -92.5) -> (-37.5, -92.5)
  line L596 (-42.5, -97.5) -> (-42.5, -92.5)
  line L597 (-47.5, -97.5) -> (-42.5, -97.5)
  line L598 (-47.5, -92.5) -> (-47.5, -97.5)
  line L599 (-42.5, -92.5) -> (-47.5, -92.5)
  line L600 (-52.5, -97.5) -> (-52.5, -92.5)
  line L601 (-57.5, -97.5) -> (-52.5, -97.5)
  line L602 (-57.5, -92.5) -> (-57.5, -97.5)
  line L603 (-52.5, -92.5) -> (-57.5, -92.5)
  line L604 (-62.5, -97.5) -> (-62.5, -92.5)
  line L605 (-67.5, -97.5) -> (-62.5, -97.5)
  line L606 (-67.5, -92.5) -> (-67.5, -97.5)
  line L607 (-62.5, -92.5) -> (-67.5, -92.5)
  line L608 (-72.5, -97.5) -> (-72.5, -92.5)
  line L609 (-77.5, -97.5) -> (-72.5, -97.5)
  line L610 (-77.5, -92.5) -> (-77.5, -97.5)
  line L611 (-72.5, -92.5) -> (-77.5, -92.5)
  line L612 (-82.5, -97.5) -> (-82.5, -92.5)
  line L613 (-87.5, -97.5) -> (-82.5, -97.5)
  line L614 (-87.5, -92.5) -> (-87.5, -97.5)
  line L615 (-82.5, -92.5) -> (-87.5, -92.5)
  line L616 (-92.5, -97.5) -> (-92.5, -92.5)
  line L617 (-97.5, -97.5) -> (-92.5, -97.5)
  line L618 (-97.5, -92.5) -> (-97.5, -97.5)
  line L619 (-92.5, -92.5) -> (-97.5, -92.5)
  line L620 (-102.5, -97.5) -> (-102.5, -92.5)
  line L621 (-107.5, -97.5) -> (-102.5, -97.5)
  line L622 (-107.5, -92.5) -> (-107.5, -97.5)
  line L623 (-102.5, -92.5) -> (-107.5, -92.5)
  line L624 (-112.5, -97.5) -> (-112.5, -92.5)
  line L625 (-117.5, -97.5) -> (-112.5, -97.5)
  line L626 (-117.5, -92.5) -> (-117.5, -97.5)
  line L627 (-112.5, -92.5) -> (-117.5, -92.5)
  line L628 (-122.5, -97.5) -> (-122.5, -92.5)
  line L629 (-127.5, -97.5) -> (-122.5, -97.5)
  line L630 (-127.5, -92.5) -> (-127.5, -97.5)
  line L631 (-122.5, -92.5) -> (-127.5, -92.5)
  line L632 (-132.5, -97.5) -> (-132.5, -92.5)
  line L633 (-137.5, -97.5) -> (-132.5, -97.5)
  line L634 (-137.5, -92.5) -> (-137.5, -97.5)
  line L635 (-132.5, -92.5) -> (-137.5, -92.5)
  line L636 (-142.5, -97.5) -> (-142.5, -92.5)
  line L637 (-147.5, -97.5) -> (-142.5, -97.5)
  line L638 (-147.5, -92.5) -> (-147.5, -97.5)
  line L639 (-142.5, -92.5) -> (-147.5, -92.5)
  line L640 (-152.5, -97.5) -> (-152.5, -92.5)
  line L641 (-157.5, -97.5) -> (-152.5, -97.5)
  line L642 (-157.5, -92.5) -> (-157.5, -97.5)
  line L643 (-152.5, -92.5) -> (-157.5, -92.5)
  line L644 (-2.5, -107.5) -> (-2.5, -102.5)
  line L645 (-7.5, -107.5) -> (-2.5, -107.5)
  line L646 (-7.5, -102.5) -> (-7.5, -107.5)
  line L647 (-2.5, -102.5) -> (-7.5, -102.5)
  line L648 (-12.5, -107.5) -> (-12.5, -102.5)
  line L649 (-17.5, -107.5) -> (-12.5, -107.5)
  line L650 (-17.5, -102.5) -> (-17.5, -107.5)
  line L651 (-12.5, -102.5) -> (-17.5, -102.5)
  line L652 (-22.5, -107.5) -> (-22.5, -102.5)
  line L653 (-27.5, -107.5) -> (-22.5, -107.5)
  line L654 (-27.5, -102.5) -> (-27.5, -107.5)
  line L655 (-22.5, -102.5) -> (-27.5, -102.5)
  line L656 (-32.5, -107.5) -> (-32.5, -102.5)
  line L657 (-37.5, -107.5) -> (-32.5, -107.5)
  line L658 (-37.5, -102.5) -> (-37.5, -107.5)
  line L659 (-32.5, -102.5) -> (-37.5, -102.5)
  line L660 (-42.5, -107.5) -> (-42.5, -102.5)
  line L661 (-47.5, -107.5) -> (-42.5, -107.5)
  line L662 (-47.5, -102.5) -> (-47.5, -107.5)
  line L663 (-42.5, -102.5) -> (-47.5, -102.5)
  line L664 (-52.5, -107.5) -> (-52.5, -102.5)
  line L665 (-57.5, -107.5) -> (-52.5, -107.5)
  line L666 (-57.5, -102.5) -> (-57.5, -107.5)
  line L667 (-52.5, -102.5) -> (-57.5, -102.5)
  line L668 (-62.5, -107.5) -> (-62.5, -102.5)
  line L669 (-67.5, -107.5) -> (-62.5, -107.5)
  line L670 (-67.5, -102.5) -> (-67.5, -107.5)
  line L671 (-62.5, -102.5) -> (-67.5, -102.5)
  line L672 (-72.5, -107.5) -> (-72.5, -102.5)
  line L673 (-77.5, -107.5) -> (-72.5, -107.5)
  line L674 (-77.5, -102.5) -> (-77.5, -107.5)
  line L675 (-72.5, -102.5) -> (-77.5, -102.5)
  line L676 (-82.5, -107.5) -> (-82.5, -102.5)
  line L677 (-87.5, -107.5) -> (-82.5, -107.5)
  line L678 (-87.5, -102.5) -> (-87.5, -107.5)
  line L679 (-82.5, -102.5) -> (-87.5, -102.5)
  line L680 (-92.5, -107.5) -> (-92.5, -102.5)
  line L681 (-97.5, -107.5) -> (-92.5, -107.5)
  line L682 (-97.5, -102.5) -> (-97.5, -107.5)
  line L683 (-92.5, -102.5) -> (-97.5, -102.5)
  line L684 (-102.5, -107.5) -> (-102.5, -102.5)
  line L685 (-107.5, -107.5) -> (-102.5, -107.5)
  line L686 (-107.5, -102.5) -> (-107.5, -107.5)
  line L687 (-102.5, -102.5) -> (-107.5, -102.5)
  line L688 (-112.5, -107.5) -> (-112.5, -102.5)
  line L689 (-117.5, -107.5) -> (-112.5, -107.5)
  line L690 (-117.5, -102.5) -> (-117.5, -107.5)
  line L691 (-112.5, -102.5) -> (-117.5, -102.5)
  line L692 (-122.5, -107.5) -> (-122.5, -102.5)
  line L693 (-127.5, -107.5) -> (-122.5, -107.5)
  line L694 (-127.5, -102.5) -> (-127.5, -107.5)
  line L695 (-122.5, -102.5) -> (-127.5, -102.5)
  line L696 (-132.5, -107.5) -> (-132.5, -102.5)
  line L697 (-137.5, -107.5) -> (-132.5, -107.5)
  line L698 (-137.5, -102.5) -> (-137.5, -107.5)
  line L699 (-132.5, -102.5) -> (-137.5, -102.5)
  line L700 (-142.5, -107.5) -> (-142.5, -102.5)
  line L701 (-147.5, -107.5) -> (-142.5, -107.5)
  line L702 (-147.5, -102.5) -> (-147.5, -107.5)
  line L703 (-142.5, -102.5) -> (-147.5, -102.5)
  line L704 (-152.5, -107.5) -> (-152.5, -102.5)
  line L705 (-157.5, -107.5) -> (-152.5, -107.5)
  line L706 (-157.5, -102.5) -> (-157.5, -107.5)
  line L707 (-152.5, -102.5) -> (-157.5, -102.5)
  line L708 (-2.5, -117.5) -> (-2.5, -112.5)
  line L709 (-7.5, -117.5) -> (-2.5, -117.5)
  line L710 (-7.5, -112.5) -> (-7.5, -117.5)
  line L711 (-2.5, -112.5) -> (-7.5, -112.5)
  line L712 (-12.5, -117.5) -> (-12.5, -112.5)
  line L713 (-17.5, -117.5) -> (-12.5, -117.5)
  line L714 (-17.5, -112.5) -> (-17.5, -117.5)
  line L715 (-12.5, -112.5) -> (-17.5, -112.5)
  line L716 (-22.5, -117.5) -> (-22.5, -112.5)
  line L717 (-27.5, -117.5) -> (-22.5, -117.5)
  line L718 (-27.5, -112.5) -> (-27.5, -117.5)
  line L719 (-22.5, -112.5) -> (-27.5, -112.5)
  line L720 (-32.5, -117.5) -> (-32.5, -112.5)
  line L721 (-37.5, -117.5) -> (-32.5, -117.5)
  line L722 (-37.5, -112.5) -> (-37.5, -117.5)
  line L723 (-32.5, -112.5) -> (-37.5, -112.5)
  line L724 (-42.5, -117.5) -> (-42.5, -112.5)
  line L725 (-47.5, -117.5) -> (-42.5, -117.5)
  line L726 (-47.5, -112.5) -> (-47.5, -117.5)
  line L727 (-42.5, -112.5) -> (-47.5, -112.5)
  line L728 (-52.5, -117.5) -> (-52.5, -112.5)
  line L729 (-57.5, -117.5) -> (-52.5, -117.5)
  line L730 (-57.5, -112.5) -> (-57.5, -117.5)
  line L731 (-52.5, -112.5) -> (-57.5, -112.5)
  line L732 (-62.5, -117.5) -> (-62.5, -112.5)
  line L733 (-67.5, -117.5) -> (-62.5, -117.5)
  line L734 (-67.5, -112.5) -> (-67.5, -117.5)
  line L735 (-62.5, -112.5) -> (-67.5, -112.5)
  line L736 (-72.5, -117.5) -> (-72.5, -112.5)
  line L737 (-77.5, -117.5) -> (-72.5, -117.5)
  line L738 (-77.5, -112.5) -> (-77.5, -117.5)
  line L739 (-72.5, -112.5) -> (-77.5, -112.5)
  line L740 (-82.5, -117.5) -> (-82.5, -112.5)
  line L741 (-87.5, -117.5) -> (-82.5, -117.5)
  line L742 (-87.5, -112.5) -> (-87.5, -117.5)
  line L743 (-82.5, -112.5) -> (-87.5, -112.5)
  line L744 (-92.5, -117.5) -> (-92.5, -112.5)
  line L745 (-97.5, -117.5) -> (-92.5, -117.5)
  line L746 (-97.5, -112.5) -> (-97.5, -117.5)
  line L747 (-92.5, -112.5) -> (-97.5, -112.5)
  line L748 (-102.5, -117.5) -> (-102.5, -112.5)
  line L749 (-107.5, -117.5) -> (-102.5, -117.5)
  line L750 (-107.5, -112.5) -> (-107.5, -117.5)
  line L751 (-102.5, -112.5) -> (-107.5, -112.5)
  line L752 (-112.5, -117.5) -> (-112.5, -112.5)
  line L753 (-117.5, -117.5) -> (-112.5, -117.5)
  line L754 (-117.5, -112.5) -> (-117.5, -117.5)
  line L755 (-112.5, -112.5) -> (-117.5, -112.5)
  line L756 (-122.5, -117.5) -> (-122.5, -112.5)
  line L757 (-127.5, -117.5) -> (-122.5, -117.5)
  line L758 (-127.5, -112.5) -> (-127.5, -117.5)
  line L759 (-122.5, -112.5) -> (-127.5, -112.5)
  line L760 (-132.5, -117.5) -> (-132.5, -112.5)
  line L761 (-137.5, -117.5) -> (-132.5, -117.5)
  line L762 (-137.5, -112.5) -> (-137.5, -117.5)
  line L763 (-132.5, -112.5) -> (-137.5, -112.5)
  line L764 (-142.5, -117.5) -> (-142.5, -112.5)
  line L765 (-147.5, -117.5) -> (-142.5, -117.5)
  line L766 (-147.5, -112.5) -> (-147.5, -117.5)
  line L767 (-142.5, -112.5) -> (-147.5, -112.5)
  line L768 (-152.5, -117.5) -> (-152.5, -112.5)
  line L769 (-157.5, -117.5) -> (-152.5, -117.5)
  line L770 (-157.5, -112.5) -> (-157.5, -117.5)
  line L771 (-152.5, -112.5) -> (-157.5, -112.5)
  line L772 (-2.5, -127.5) -> (-2.5, -122.5)
  line L773 (-7.5, -127.5) -> (-2.5, -127.5)
  line L774 (-7.5, -122.5) -> (-7.5, -127.5)
  line L775 (-2.5, -122.5) -> (-7.5, -122.5)
  line L776 (-12.5, -127.5) -> (-12.5, -122.5)
  line L777 (-17.5, -127.5) -> (-12.5, -127.5)
  line L778 (-17.5, -122.5) -> (-17.5, -127.5)
  line L779 (-12.5, -122.5) -> (-17.5, -122.5)
  line L780 (-22.5, -127.5) -> (-22.5, -122.5)
  line L781 (-27.5, -127.5) -> (-22.5, -127.5)
  line L782 (-27.5, -122.5) -> (-27.5, -127.5)
  line L783 (-22.5, -122.5) -> (-27.5, -122.5)
  line L784 (-32.5, -127.5) -> (-32.5, -122.5)
  line L785 (-37.5, -127.5) -> (-32.5, -127.5)
  line L786 (-37.5, -122.5) -> (-37.5, -127.5)
  line L787 (-32.5, -122.5) -> (-37.5, -122.5)
  line L788 (-42.5, -127.5) -> (-42.5, -122.5)
  line L789 (-47.5, -127.5) -> (-42.5, -127.5)
  line L790 (-47.5, -122.5) -> (-47.5, -127.5)
  line L791 (-42.5, -122.5) -> (-47.5, -122.5)
  line L792 (-52.5, -127.5) -> (-52.5, -122.5)
  line L793 (-57.5, -127.5) -> (-52.5, -127.5)
  line L794 (-57.5, -122.5) -> (-57.5, -127.5)
  line L795 (-52.5, -122.5) -> (-57.5, -122.5)
  line L796 (-62.5, -127.5) -> (-62.5, -122.5)
  line L797 (-67.5, -127.5) -> (-62.5, -127.5)
  line L798 (-67.5, -122.5) -> (-67.5, -127.5)
  line L799 (-62.5, -122.5) -> (-67.5, -122.5)
  line L800 (-72.5, -127.5) -> (-72.5, -122.5)
  line L801 (-77.5, -127.5) -> (-72.5, -127.5)
  line L802 (-77.5, -122.5) -> (-77.5, -127.5)
  line L803 (-72.5, -122.5) -> (-77.5, -122.5)
  line L804 (-82.5, -127.5) -> (-82.5, -122.5)
  line L805 (-87.5, -127.5) -> (-82.5, -127.5)
  line L806 (-87.5, -122.5) -> (-87.5, -127.5)
  line L807 (-82.5, -122.5) -> (-87.5, -122.5)
  line L808 (-92.5, -127.5) -> (-92.5, -122.5)
  line L809 (-97.5, -127.5) -> (-92.5, -127.5)
  line L810 (-97.5, -122.5) -> (-97.5, -127.5)
  line L811 (-92.5, -122.5) -> (-97.5, -122.5)
  line L812 (-102.5, -127.5) -> (-102.5, -122.5)
  line L813 (-107.5, -127.5) -> (-102.5, -127.5)
  line L814 (-107.5, -122.5) -> (-107.5, -127.5)
  line L815 (-102.5, -122.5) -> (-107.5, -122.5)
  line L816 (-112.5, -127.5) -> (-112.5, -122.5)
  line L817 (-117.5, -127.5) -> (-112.5, -127.5)
  line L818 (-117.5, -122.5) -> (-117.5, -127.5)
  line L819 (-112.5, -122.5) -> (-117.5, -122.5)
  line L820 (-122.5, -127.5) -> (-122.5, -122.5)
  line L821 (-127.5, -127.5) -> (-122.5, -127.5)
  line L822 (-127.5, -122.5) -> (-127.5, -127.5)
  line L823 (-122.5, -122.5) -> (-127.5, -122.5)
  line L824 (-132.5, -127.5) -> (-132.5, -122.5)
  line L825 (-137.5, -127.5) -> (-132.5, -127.5)
  line L826 (-137.5, -122.5) -> (-137.5, -127.5)
  line L827 (-132.5, -122.5) -> (-137.5, -122.5)
  line L828 (-142.5, -127.5) -> (-142.5, -122.5)
  line L829 (-147.5, -127.5) -> (-142.5, -127.5)
  line L830 (-147.5, -122.5) -> (-147.5, -127.5)
  line L831 (-142.5, -122.5) -> (-147.5, -122.5)
  line L832 (-152.5, -127.5) -> (-152.5, -122.5)
  line L833 (-157.5, -127.5) -> (-152.5, -127.5)
  line L834 (-157.5, -122.5) -> (-157.5, -127.5)
  line L835 (-152.5, -122.5) -> (-157.5, -122.5)
  line L836 (-2.5, -137.5) -> (-2.5, -132.5)
  line L837 (-7.5, -137.5) -> (-2.5, -137.5)
  line L838 (-7.5, -132.5) -> (-7.5, -137.5)
  line L839 (-2.5, -132.5) -> (-7.5, -132.5)
  line L840 (-12.5, -137.5) -> (-12.5, -132.5)
  line L841 (-17.5, -137.5) -> (-12.5, -137.5)
  line L842 (-17.5, -132.5) -> (-17.5, -137.5)
  line L843 (-12.5, -132.5) -> (-17.5, -132.5)
  line L844 (-22.5, -137.5) -> (-22.5, -132.5)
  line L845 (-27.5, -137.5) -> (-22.5, -137.5)
  line L846 (-27.5, -132.5) -> (-27.5, -137.5)
  line L847 (-22.5, -132.5) -> (-27.5, -132.5)
  line L848 (-32.5, -137.5) -> (-32.5, -132.5)
  line L849 (-37.5, -137.5) -> (-32.5, -137.5)
  line L850 (-37.5, -132.5) -> (-37.5, -137.5)
  line L851 (-32.5, -132.5) -> (-37.5, -132.5)
  line L852 (-42.5, -137.5) -> (-42.5, -132.5)
  line L853 (-47.5, -137.5) -> (-42.5, -137.5)
  line L854 (-47.5, -132.5) -> (-47.5, -137.5)
  line L855 (-42.5, -132.5) -> (-47.5, -132.5)
  line L856 (-52.5, -137.5) -> (-52.5, -132.5)
  line L857 (-57.5, -137.5) -> (-52.5, -137.5)
  line L858 (-57.5, -132.5) -> (-57.5, -137.5)
  line L859 (-52.5, -132.5) -> (-57.5, -132.5)
  line L860 (-62.5, -137.5) -> (-62.5, -132.5)
  line L861 (-67.5, -137.5) -> (-62.5, -137.5)
  line L862 (-67.5, -132.5) -> (-67.5, -137.5)
  line L863 (-62.5, -132.5) -> (-67.5, -132.5)
  line L864 (-72.5, -137.5) -> (-72.5, -132.5)
  line L865 (-77.5, -137.5) -> (-72.5, -137.5)
  line L866 (-77.5, -132.5) -> (-77.5, -137.5)
  line L867 (-72.5, -132.5) -> (-77.5, -132.5)
  line L868 (-82.5, -137.5) -> (-82.5, -132.5)
  line L869 (-87.5, -137.5) -> (-82.5, -137.5)
  line L870 (-87.5, -132.5) -> (-87.5, -137.5)
  line L871 (-82.5, -132.5) -> (-87.5, -132.5)
  line L872 (-92.5, -137.5) -> (-92.5, -132.5)
  line L873 (-97.5, -137.5) -> (-92.5, -137.5)
  line L874 (-97.5, -132.5) -> (-97.5, -137.5)
  line L875 (-92.5, -132.5) -> (-97.5, -132.5)
  line L876 (-102.5, -137.5) -> (-102.5, -132.5)
  line L877 (-107.5, -137.5) -> (-102.5, -137.5)
  line L878 (-107.5, -132.5) -> (-107.5, -137.5)
  line L879 (-102.5, -132.5) -> (-107.5, -132.5)
  line L880 (-112.5, -137.5) -> (-112.5, -132.5)
  line L881 (-117.5, -137.5) -> (-112.5, -137.5)
  line L882 (-117.5, -132.5) -> (-117.5, -137.5)
  line L883 (-112.5, -132.5) -> (-117.5, -132.5)
  line L884 (-122.5, -137.5) -> (-122.5, -132.5)
  line L885 (-127.5, -137.5) -> (-122.5, -137.5)
  line L886 (-127.5, -132.5) -> (-127.5, -137.5)
  line L887 (-122.5, -132.5) -> (-127.5, -132.5)
  line L888 (-132.5, -137.5) -> (-132.5, -132.5)
  line L889 (-137.5, -137.5) -> (-132.5, -137.5)
  line L890 (-137.5, -132.5) -> (-137.5, -137.5)
  line L891 (-132.5, -132.5) -> (-137.5, -132.5)
  line L892 (-142.5, -137.5) -> (-142.5, -132.5)
  line L893 (-147.5, -137.5) -> (-142.5, -137.5)
  line L894 (-147.5, -132.5) -> (-147.5, -137.5)
  line L895 (-142.5, -132.5) -> (-147.5, -132.5)
  line L896 (-152.5, -137.5) -> (-152.5, -132.5)
  line L897 (-157.5, -137.5) -> (-152.5, -137.5)
  line L898 (-157.5, -132.5) -> (-157.5, -137.5)
  line L899 (-152.5, -132.5) -> (-157.5, -132.5)
  line L900 (-2.5, -147.5) -> (-2.5, -142.5)
  line L901 (-7.5, -147.5) -> (-2.5, -147.5)
  line L902 (-7.5, -142.5) -> (-7.5, -147.5)
  line L903 (-2.5, -142.5) -> (-7.5, -142.5)
  line L904 (-12.5, -147.5) -> (-12.5, -142.5)
  line L905 (-17.5, -147.5) -> (-12.5, -147.5)
  line L906 (-17.5, -142.5) -> (-17.5, -147.5)
  line L907 (-12.5, -142.5) -> (-17.5, -142.5)
  line L908 (-22.5, -147.5) -> (-22.5, -142.5)
  line L909 (-27.5, -147.5) -> (-22.5, -147.5)
  line L910 (-27.5, -142.5) -> (-27.5, -147.5)
  line L911 (-22.5, -142.5) -> (-27.5, -142.5)
  line L912 (-32.5, -147.5) -> (-32.5, -142.5)
  line L913 (-37.5, -147.5) -> (-32.5, -147.5)
  line L914 (-37.5, -142.5) -> (-37.5, -147.5)
  line L915 (-32.5, -142.5) -> (-37.5, -142.5)
  line L916 (-42.5, -147.5) -> (-42.5, -142.5)
  line L917 (-47.5, -147.5) -> (-42.5, -147.5)
  line L918 (-47.5, -142.5) -> (-47.5, -147.5)
  line L919 (-42.5, -142.5) -> (-47.5, -142.5)
  line L920 (-52.5, -147.5) -> (-52.5, -142.5)
  line L921 (-57.5, -147.5) -> (-52.5, -147.5)
  line L922 (-57.5, -142.5) -> (-57.5, -147.5)
  line L923 (-52.5, -142.5) -> (-57.5, -142.5)
  line L924 (-62.5, -147.5) -> (-62.5, -142.5)
  line L925 (-67.5, -147.5) -> (-62.5, -147.5)
  line L926 (-67.5, -142.5) -> (-67.5, -147.5)
  line L927 (-62.5, -142.5) -> (-67.5, -142.5)
  line L928 (-72.5, -147.5) -> (-72.5, -142.5)
  line L929 (-77.5, -147.5) -> (-72.5, -147.5)
  line L930 (-77.5, -142.5) -> (-77.5, -147.5)
  line L931 (-72.5, -142.5) -> (-77.5, -142.5)
  line L932 (-82.5, -147.5) -> (-82.5, -142.5)
  line L933 (-87.5, -147.5) -> (-82.5, -147.5)
  line L934 (-87.5, -142.5) -> (-87.5, -147.5)
  line L935 (-82.5, -142.5) -> (-87.5, -142.5)
  line L936 (-92.5, -147.5) -> (-92.5, -142.5)
  line L937 (-97.5, -147.5) -> (-92.5, -147.5)
  line L938 (-97.5, -142.5) -> (-97.5, -147.5)
  line L939 (-92.5, -142.5) -> (-97.5, -142.5)
  line L940 (-102.5, -147.5) -> (-102.5, -142.5)
  line L941 (-107.5, -147.5) -> (-102.5, -147.5)
  line L942 (-107.5, -142.5) -> (-107.5, -147.5)
  line L943 (-102.5, -142.5) -> (-107.5, -142.5)
  line L944 (-112.5, -147.5) -> (-112.5, -142.5)
  line L945 (-117.5, -147.5) -> (-112.5, -147.5)
  line L946 (-117.5, -142.5) -> (-117.5, -147.5)
  line L947 (-112.5, -142.5) -> (-117.5, -142.5)
  line L948 (-122.5, -147.5) -> (-122.5, -142.5)
  line L949 (-127.5, -147.5) -> (-122.5, -147.5)
  line L950 (-127.5, -142.5) -> (-127.5, -147.5)
  line L951 (-122.5, -142.5) -> (-127.5, -142.5)
  line L952 (-132.5, -147.5) -> (-132.5, -142.5)
  line L953 (-137.5, -147.5) -> (-132.5, -147.5)
  line L954 (-137.5, -142.5) -> (-137.5, -147.5)
  line L955 (-132.5, -142.5) -> (-137.5, -142.5)
  line L956 (-142.5, -147.5) -> (-142.5, -142.5)
  line L957 (-147.5, -147.5) -> (-142.5, -147.5)
  line L958 (-147.5, -142.5) -> (-147.5, -147.5)
  line L959 (-142.5, -142.5) -> (-147.5, -142.5)
  line L960 (-152.5, -147.5) -> (-152.5, -142.5)
  line L961 (-157.5, -147.5) -> (-152.5, -147.5)
  line L962 (-157.5, -142.5) -> (-157.5, -147.5)
  line L963 (-152.5, -142.5) -> (-157.5, -142.5)
  line L964 (-2.5, -157.5) -> (-2.5, -152.5)
  line L965 (-7.5, -157.5) -> (-2.5, -157.5)
  line L966 (-7.5, -152.5) -> (-7.5, -157.5)
  line L967 (-2.5, -152.5) -> (-7.5, -152.5)
  line L968 (-12.5, -157.5) -> (-12.5, -152.5)
  line L969 (-17.5, -157.5) -> (-12.5, -157.5)
  line L970 (-17.5, -152.5) -> (-17.5, -157.5)
  line L971 (-12.5, -152.5) -> (-17.5, -152.5)
  line L972 (-22.5, -157.5) -> (-22.5, -152.5)
  line L973 (-27.5, -157.5) -> (-22.5, -157.5)
  line L974 (-27.5, -152.5) -> (-27.5, -157.5)
  line L975 (-22.5, -152.5) -> (-27.5, -152.5)
  line L976 (-32.5, -157.5) -> (-32.5, -152.5)
  line L977 (-37.5, -157.5) -> (-32.5, -157.5)
  line L978 (-37.5, -152.5) -> (-37.5, -157.5)
  line L979 (-32.5, -152.5) -> (-37.5, -152.5)
  line L980 (-42.5, -157.5) -> (-42.5, -152.5)
  line L981 (-47.5, -157.5) -> (-42.5, -157.5)
  line L982 (-47.5, -152.5) -> (-47.5, -157.5)
  line L983 (-42.5, -152.5) -> (-47.5, -152.5)
  line L984 (-52.5, -157.5) -> (-52.5, -152.5)
  line L985 (-57.5, -157.5) -> (-52.5, -157.5)
  line L986 (-57.5, -152.5) -> (-57.5, -157.5)
  line L987 (-52.5, -152.5) -> (-57.5, -152.5)
  line L988 (-62.5, -157.5) -> (-62.5, -152.5)
  line L989 (-67.5, -157.5) -> (-62.5, -157.5)
  line L990 (-67.5, -152.5) -> (-67.5, -157.5)
  line L991 (-62.5, -152.5) -> (-67.5, -152.5)
  line L992 (-72.5, -157.5) -> (-72.5, -152.5)
  line L993 (-77.5, -157.5) -> (-72.5, -157.5)
  line L994 (-77.5, -152.5) -> (-77.5, -157.5)
  line L995 (-72.5, -152.5) -> (-77.5, -152.5)
  line L996 (-82.5, -157.5) -> (-82.5, -152.5)
  line L997 (-87.5, -157.5) -> (-82.5, -157.5)
  line L998 (-87.5, -152.5) -> (-87.5, -157.5)
  line L999 (-82.5, -152.5) -> (-87.5, -152.5)
  line L1000 (-92.5, -157.5) -> (-92.5, -152.5)
  line L1001 (-97.5, -157.5) -> (-92.5, -157.5)
  line L1002 (-97.5, -152.5) -> (-97.5, -157.5)
  line L1003 (-92.5, -152.5) -> (-97.5, -152.5)
  line L1004 (-102.5, -157.5) -> (-102.5, -152.5)
  line L1005 (-107.5, -157.5) -> (-102.5, -157.5)
  line L1006 (-107.5, -152.5) -> (-107.5, -157.5)
  line L1007 (-102.5, -152.5) -> (-107.5, -152.5)
  line L1008 (-112.5, -157.5) -> (-112.5, -152.5)
  line L1009 (-117.5, -157.5) -> (-112.5, -157.5)
  line L1010 (-117.5, -152.5) -> (-117.5, -157.5)
  line L1011 (-112.5, -152.5) -> (-117.5, -152.5)
  line L1012 (-122.5, -157.5) -> (-122.5, -152.5)
  line L1013 (-127.5, -157.5) -> (-122.5, -157.5)
  line L1014 (-127.5, -152.5) -> (-127.5, -157.5)
  line L1015 (-122.5, -152.5) -> (-127.5, -152.5)
  line L1016 (-132.5, -157.5) -> (-132.5, -152.5)
  line L1017 (-137.5, -157.5) -> (-132.5, -157.5)
  line L1018 (-137.5, -152.5) -> (-137.5, -157.5)
  line L1019 (-132.5, -152.5) -> (-137.5, -152.5)
  line L1020 (-142.5, -157.5) -> (-142.5, -152.5)
  line L1021 (-147.5, -157.5) -> (-142.5, -157.5)
  line L1022 (-147.5, -152.5) -> (-147.5, -157.5)
  line L1023 (-142.5, -152.5) -> (-147.5, -152.5)
  line L1024 (-152.5, -157.5) -> (-152.5, -152.5)
  line L1025 (-157.5, -157.5) -> (-152.5, -157.5)
  line L1026 (-157.5, -152.5) -> (-157.5, -157.5)
  line L1027 (-152.5, -152.5) -> (-157.5, -152.5)
  line L1028 (-9, -2.5) -> (-11, -2.5)
  line L1029 (-11, -2.5) -> (-11, -5)
  line L1030 (-11, -5) -> (-9, -5)
  line L1031 (-9, -5) -> (-9, -2.5)
  line L1032 (-21, -5) -> (-19, -5)
  line L1033 (-19, -5) -> (-19, -2.5)
  line L1034 (-21, -2.5) -> (-21, -5)
  line L1035 (-19, -2.5) -> (-21, -2.5)
  line L1036 (-31, -5) -> (-29, -5)
  line L1037 (-29, -5) -> (-29, -2.5)
  line L1038 (-31, -2.5) -> (-31, -5)
  line L1039 (-29, -2.5) -> (-31, -2.5)
  line L1040 (-41, -5) -> (-39, -5)
  line L1041 (-39, -5) -> (-39, -2.5)
  line L1042 (-41, -2.5) -> (-41, -5)
  line L1043 (-39, -2.5) -> (-41, -2.5)
  line L1044 (-51, -5) -> (-49, -5)
  line L1045 (-49, -5) -> (-49, -2.5)
  line L1046 (-51, -2.5) -> (-51, -5)
  line L1047 (-49, -2.5) -> (-51, -2.5)
  line L1048 (-61, -5) -> (-59, -5)
  line L1049 (-59, -5) -> (-59, -2.5)
  line L1050 (-61, -2.5) -> (-61, -5)
  line L1051 (-59, -2.5) -> (-61, -2.5)
  line L1052 (-71, -5) -> (-69, -5)
  line L1053 (-69, -5) -> (-69, -2.5)
  line L1054 (-71, -2.5) -> (-71, -5)
  line L1055 (-69, -2.5) -> (-71, -2.5)
  line L1056 (-81, -5) -> (-79, -5)
  line L1057 (-79, -5) -> (-79, -2.5)
  line L1058 (-81, -2.5) -> (-81, -5)
  line L1059 (-79, -2.5) -> (-81, -2.5)
  line L1060 (-91, -5) -> (-89, -5)
  line L1061 (-89, -5) -> (-89, -2.5)
  line L1062 (-91, -2.5) -> (-91, -5)
  line L1063 (-89, -2.5) -> (-91, -2.5)
  line L1064 (-101, -5) -> (-99, -5)
  line L1065 (-99, -5) -> (-99, -2.5)
  line L1066 (-101, -2.5) -> (-101, -5)